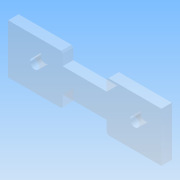
# Autodesk Inventor part: DPX Slide Jig Cover
Saved by Autodesk Inventor 2015 SP1 (Build 190203100, 203)
## iProperties
Created: 2014-11-07
Material: ACRYLIC, CLEAR
Vendor: HHMI: JFRC - ID&F
Document SubType Name: Modeling
Designer: KLOSSR
Density: 0.66 g/cm^3
Mass: 5.74639 g
Surface Area: 46.4903 cm^2
Volume: 8.70666 cm^3
Appearance: Polycarbonate - Clear
RuleStatus: InUse
AfterDocSave0: file://Part Number Cleaner
DESIGN DEPARTMENT: HHMI: JFRC - ID&F
ALTERED ITEM PART NUMBER: N/A
ALTERED ITEM VENDOR: N/A
ALTERED ITEM DESCRIPTION: N/A
Author: KLOSSR
Revision Number: 0
Autodesk Inventor part; units mm, degrees
ref_plane "YZ Plane" through (0, 0, 0) normal (1, 0, 0) x (0, 1, 0)
ref_plane "XZ Plane" through (0, 0, 0) normal (0, 1, 0) x (-1, 0, 0)
ref_plane "XY Plane" through (0, 0, 0) normal (0, 0, 1) x (1, 0, 0)
sketch "Sketch1" plane through (0, 0, 0) normal (0, 0, 1) x (1, 0, 0)
  line L0 (-38.9255, 12.5476) -> (38.9255, 12.5476)
  line L1 (38.9255, 12.5476) -> (38.9255, -12.5476)
  line L2 (38.9255, -12.5476) -> (-38.9255, -12.5476)
  line L3 (-38.9255, -12.5476) -> (-38.9255, 12.5476)
  point P0 (0, 0)
  point P1 (38.9255, 0)
  point P2 (0, 12.5476)
  dimension "d0" = 77.851
  dimension "d1" = 25.0952
  constraints: 8 end point, 2 midpoint, 2 parallel, 1 horizontal, 1 horizontal alignment, 1 perpendicular, 1 vertical alignment
  measures "d0" distance of L0.start L0.end
  measures "d1" distance of L0.end L1.end
extrude "Extrusion1" add sketch "Sketch1" against normal blind 5.334
sketch "Sketch2" plane through (0, 0, 0) normal (0, 0, 1) x (1, 0, 0)
  line L0 (-38.9255, 12.5476) -> (38.9255, 12.5476) projected
  line L1 (38.9255, -12.5476) -> (-38.9255, -12.5476) projected
  line L2 (-11.176, -6.1976) -> (11.176, -6.1976)
  line L3 (11.176, -6.1976) -> (11.176, -12.5476)
  line L4 (11.176, -12.5476) -> (-11.176, -12.5476)
  line L5 (-11.176, -12.5476) -> (-11.176, -6.1976)
  point P0 (0, 0)
  point P1 (0, -6.1976)
  point P2 (0, 12.5476)
  dimension "d4" = 22.352
  dimension "d5" = 6.35
  constraints: 8 end point, 2 midpoint, 2 parallel, 1 collinear, 1 horizontal, 1 perpendicular, 1 vertical alignment
  measures "d4" distance of L2.start L2.end
  measures "d5" distance of L2.end L3.end
extrude "Extrusion2" cut sketch "Sketch2" against normal blind 25.4
mirror "Mirror1" about plane through (0, 0, 0) normal (0, 1, 0) of "Extrusion2"
sketch "Sketch3" plane through (0, 0, 0) normal (0, 0, 1) x (1, 0, 0)
  line L0 (-54.4957, 0) -> (54.4957, 0) projected
  line L1 (0, 17.5666) -> (0, -17.5666) projected
  point P0 (0, 0)
  point P1 (-25.4, 0)
  dimension "d8" = 25.4
  constraints: 1 point on line
  measures "d8" distance from line of point (-25.4, 0) L1
hole "Hole1" at (-25.4, 0, 0) direction (0, 0, -1) diameter 4.8006 end through all
mirror "Mirror2" about plane through (0, 0, 0) normal (1, 0, 0) of "Hole1"
chamfer "Chamfer1" distance 0.8128 angle 45 4 edges at (11.176, 12.5476, -2.667) (-11.176, 12.5476, -2.667) (11.176, -12.5476, -2.667) (-11.176, -12.5476, -2.667)
body "Solid1"
